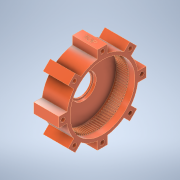
# Autodesk Inventor part: Gear_Box_Chasis_Lvl_1
Saved by Autodesk Inventor 2022 (Build 260153000, 153)
## iProperties
CustomPartVersion: 1
Created: 2022-04-22
Part Number: Gear_Box_Chasis_Lvl_1
Material: ABS Plastic
Document SubType Name: Modeling
Designer: Mlees
Categories: <?xml version="1.0" encoding="UTF-16"?> <MemberInstance><Categories><FamilyTemplate><FamilyTemplateParameter ValueType="xs:double" Id="1" ObjectReferenceKey="da_z" ObjectType="kUserParameterObject"/><FamilyTemplateParameter ValueType="xs:double" Id="2" ObjectReferenceKey="da_b" ObjectType="kUserParameterObject"/><FamilyTemplateParameter ValueType="xs:double" Id="3" ObjectReferenceKey="da_beta" ObjectType="kUserParameterObject"/><FamilyTemplateParameter ValueType="xs:double" Id="4" ObjectReferenceKey="da_da" ObjectType="kUserParameterObject"/><FamilyTemplateParameter ValueType="xs:double" Id="5" ObjectReferenceKey="da_aw" ObjectType="kUserParameterObject"/><FamilyTemplateParameter ValueType="xs:string" Id="6" ObjectReferenceKey="EAIAABAAAACIAQAAAAAAAIAAAAAAAAAA" ObjectType="83910656" SubObjectId="SurfaceGeometry"/></FamilyTemplate><ParamToTemplateMap><ParamToTemplate CategoryParameter="//CategoryParameter[@InternalName='046C89C9-8512-4d59-83FE-43B91F4F132A']" TemplateParameter="1"/><ParamToTemplate CategoryParameter="//CategoryParameter[@InternalName='2552DF32-E462-4b46-AEBF-C6C7768E72AC']" TemplateParameter="2"/><ParamToTemplate CategoryParameter="//CategoryParameter[@InternalName='C9EE641D-15FC-4fae-A226-E94C4372FDD7']" TemplateParameter="3"/><ParamToTemplate><ParamToTemplate CategoryParameter="//CategoryParameter[@InternalName='00B6519A-459B-49c7-AD84-2E56D39A5744']" ConstantValue="0.064200"/></ParamToTemplate><ParamToTemplate><ParamToTemplate CategoryParameter="//CategoryParameter[@InternalName='04B31F0E-C7A6-4894-AA32-9629BEFACF47']" ConstantValue="1.000000"/></ParamToTemplate><ParamToTemplate><ParamToTemplate CategoryParameter="//CategoryParameter[@InternalName='43CBEC2E-7847-49e7-A936-2F7889FCB2D9']" ConstantValue="0.250000"/></ParamToTemplate><ParamToTemplate><ParamToTemplate CategoryParameter="//CategoryParameter[@InternalName='B1EFC894-105D-4ebd-86BF-FA20ED196853']" ConstantValue="0.333500"/></ParamToTemplate><ParamToTemplate><ParamToTemplate CategoryParameter="//CategoryParameter[@InternalName='51175063-3D10-4879-93E8-6246FE8B403D']" ConstantValue="2060000000.000000"/></ParamToTemplate><ParamToTemplate><ParamToTemplate CategoryParameter="//CategoryParameter[@InternalName='A3A52E27-4454-46a9-B0BD-C932399B70AF']" ConstantValue="0.300000"/></ParamToTemplate><ParamToTemplate><ParamToTemplate CategoryParameter="//CategoryParameter[@InternalName='91B76062-C214-41d9-B1B9-14D2AB99603D']" ConstantValue="0.055000"/></ParamToTemplate><ParamToTemplate><ParamToTemplate CategoryParameter="//CategoryParameter[@InternalName='374E806E-8B8A-4dda-A9AA-1039D6500AD2']" ConstantValue="18.181818"/></ParamToTemplate><ParamToTemplate><ParamToTemplate CategoryParameter="//CategoryParameter[@InternalName='2D373A89-B862-43d6-8D0B-0CBF12AB9F6C']" ConstantValue="0.253073"/></ParamToTemplate><ParamToTemplate CategoryParameter="//CategoryParameter[@InternalName='37777632-D6A2-4fac-9D53-DB8ACD95C989']" TemplateParameter="4"/><ParamToTemplate CategoryParameter="//CategoryParameter[@InternalName='FD1017F1-B727-4f7e-9707-0F86F1FF9423']" TemplateParameter="5"/><ParamToTemplate><ParamToTemplate CategoryParameter="//CategoryParameter[@InternalName='9E1B4470-B2D3-4ff1-B813-535BB4CDF51A']" ConstantValue="3520000.000000"/></ParamToTemplate><ParamToTemplate><ParamToTemplate CategoryParameter="//CategoryParameter[@InternalName='F8452263-BFF6-458c-9FB1-07C4B99E95CD']" ConstantValue="11400000.000000"/></ParamToTemplate><ParamToTemplate><ParamToTemplate CategoryParameter="//CategoryParameter[@InternalName='3E3BB259-FD49-497f-8171-6EBC954A3479']" ConstantValue="2.000000"/></ParamToTemplate><ParamToTemplate CategoryParameter="//CategoryParameter[@InternalName='27C3BAF2-7550-4e4b-AE2C-0DB134B7D9B7']" TemplateParameter="6"/></ParamToTemplateMap><Category DisplayName="Gear" InternalName="DC85795E-93AB-48d5-8EEE-5A27447B64BD" Mnemonic="Gear"><CategoryParameter DisplayName="z" InternalName="046C89C9-8512-4d59-83FE-43B91F4F132A" Mnemonic="z"/><CategoryParameter DisplayName="b" InternalName="2552DF32-E462-4b46-AEBF-C6C7768E72AC" Mnemonic="b"/><CategoryParameter DisplayName="||b|" InternalName="C9EE641D-15FC-4fae-A226-E94C4372FDD7" Mnemonic="beta"/><CategoryParameter DisplayName="x" InternalName="00B6519A-459B-49c7-AD84-2E56D39A5744" Mnemonic="x"/><CategoryParameter DisplayName="a*" InternalName="04B31F0E-C7A6-4894-AA32-9629BEFACF47" Mnemonic="a"/><CategoryParameter DisplayName="c*" InternalName="43CBEC2E-7847-49e7-A936-2F7889FCB2D9" Mnemonic="c"/><CategoryParameter DisplayName="r|.f|*" InternalName="B1EFC894-105D-4ebd-86BF-FA20ED196853" Mnemonic="rf"/><CategoryParameter DisplayName="E" InternalName="51175063-3D10-4879-93E8-6246FE8B403D" Mnemonic="E"/><CategoryParameter DisplayName="||m|" InternalName="A3A52E27-4454-46a9-B0BD-C932399B70AF" Mnemonic="mi"/><Category DisplayName="SpurGear" InternalName="26C5A22E-A91E-4dfd-A3B3-23CCAFAE1764" Mnemonic="SpurGear"><CategoryParameter DisplayName="m" InternalName="91B76062-C214-41d9-B1B9-14D2AB99603D" Mnemonic="m"/><CategoryParameter DisplayName="P" InternalName="374E806E-8B8A-4dda-A9AA-1039D6500AD2" Mnemonic="PP"/><CategoryParameter DisplayName="||a|" InternalName="2D373A89-B862-43d6-8D0B-0CBF12AB9F6C" Mnemonic="alpha"/><CategoryParameter DisplayName="d|.a|" InternalName="37777632-D6A2-4fac-9D53-DB8ACD95C989" Mnemonic="da"/><CategoryParameter DisplayName="a|.w|" InternalName="FD1017F1-B727-4f7e-9707-0F86F1FF9423" Mnemonic="aw"/><CategoryParameter DisplayName="||s||.Flim|" InternalName="9E1B4470-B2D3-4ff1-B813-535BB4CDF51A" Mnemonic="sFlim"/><CategoryParameter DisplayName="||s||.Hlim|" InternalName="F8452263-BFF6-458c-9FB1-07C4B99E95CD" Mnemonic="sHlim"/><CategoryParameter DisplayName="type" InternalName="3E3BB259-FD49-497f-8171-6EBC954A3479" Mnemonic="type"/><Category DisplayName="InternalSpurGear" InternalName="7CF704F6-14A9-42f8-93CE-E71DF57C2B55" Mnemonic="InternalSpurGear"><CategoryParameter DisplayName="PitchDiameter" InternalName="27C3BAF2-7550-4e4b-AE2C-0DB134B7D9B7" Mnemonic="IDS_PITCHDIAM"/></Category></Category></Category></Categories></MemberInstance>
Density: 1.06 g/cm^3
Appearance: Smooth - Light Orange
Mass: 27.2175 g
Surface Area: 170.067 cm^2
Volume: 25.6769 cm^3
Author: Mlees
Autodesk Inventor part; units mm, degrees
ref_plane "YZ Plane" through (0, 0, 0) normal (1, 0, 0) x (0, 1, 0)
ref_plane "XZ Plane" through (0, 0, 0) normal (0, 1, 0) x (-1, 0, 0)
ref_plane "XY Plane" through (0, 0, 0) normal (0, 0, 1) x (1, 0, 0)
sketch "Sketch1" plane through (0, 0, 0) normal (0, 0, 1) x (1, 0, 0)
  circle A0 centre (0, 0) radius 28.6251
  dimension "d0" = 57.2502
  constraints: 1 centre point
  measures "d0" diameter of A0
extrude "Extrusion1" add sketch "Sketch1" along normal blind 8
ref_plane "Work Plane2" through (0, 0, 4) normal (0, 0, 1) x (1, 0, 0)
sketch "Sketch2" plane through (0, 0, 0) normal (0, 0, -1) x (-1, 0, 0)
  circle A0 centre (0, 0) radius 28.6251 projected
  circle A1 centre (0, 0) radius 25.3
  dimension "d3" = 50.6
  constraints: 1 centre point, 1 coincident
  measures "d3" diameter of A1
surface extrude "Pitch Diameter" sketch "Sketch2" against normal through all shown no curves A1
ref_plane "Work Plane8" through (0, 0, 0) normal (0.999417, 0.0341411, 0) x (0, 0, 1)
ref_plane "Work Plane9" through (0, 0, 0) normal (1, 0, 0) x (0, 1, 0)
spur gear teeth "Spur Gear" teeth 92 pitch diameter 50.6 tip diameter 49.6575 root diameter 52.0456 face width 8 start plane through (0, 0, 0) normal (0, 0, -1) x (-1, 0, 0)
sketch "Sketch3" plane through (0, 0, 8) normal (0, 0, 1) x (1, 0, 0)
  circle A0 centre (0, 0) radius 28.6251
  arc A1 (0.2222, -26.0219) -> (0.6358, -24.8206) centre (-6.3627, -23.0825) ccw projected
  circle A2 centre (0, 0) radius 26.0228
  constraints: 2 coincident, 1 centre point, 3 other
extrude "Extrusion2" add sketch "Sketch3" along normal blind 4
sketch "Sketch4" plane through (0, 0, 12) normal (0, 0, 1) x (1, 0, 0)
  circle A0 centre (0, 0) radius 8.5
  circle A1 centre (0, 0) radius 28.6251
  dimension "d55" = 17
  constraints: 2 centre point, 2 coincident
  measures "d55" diameter of A0
extrude "Extrusion3" add sketch "Sketch4" along normal blind 3
sketch "Sketch5" plane through (0, 0, 15) normal (0, 0, 1) x (1, 0, 0)
  circle A0 centre (0, 0) radius 8.5
  circle A1 centre (0, 0) radius 28.6251 projected
  circle A2 centre (0, 0) radius 28.6251
  line L0 (-4, 28.3442) -> (-4, 35)
  line L1 (4, 28.3442) -> (4, 35)
  line L2 (-4, 35) -> (4, 35)
  circle A3 centre (0, 31.6721) radius 1.7859
  line L3 (-27.5772, 21.9203) -> (-21.9203, 27.5772)
  circle A4 centre (-22.3956, 22.3956) radius 1.7859
  line L4 (-22.8708, 17.214) -> (-27.5772, 21.9203)
  line L5 (-17.214, 22.8708) -> (-21.9203, 27.5772)
  line L6 (-35, -4) -> (-35, 4)
  circle A5 centre (-31.6721, 0) radius 1.7859
  line L7 (-28.3442, -4) -> (-35, -4)
  line L8 (-28.3442, 4) -> (-35, 4)
  line L9 (-21.9203, -27.5772) -> (-27.5772, -21.9203)
  circle A6 centre (-22.3956, -22.3956) radius 1.7859
  line L10 (-17.214, -22.8708) -> (-21.9203, -27.5772)
  line L11 (-22.8708, -17.214) -> (-27.5772, -21.9203)
  line L12 (4, -35) -> (-4, -35)
  circle A7 centre (0, -31.6721) radius 1.7859
  line L13 (4, -28.3442) -> (4, -35)
  line L14 (-4, -28.3442) -> (-4, -35)
  line L15 (27.5772, -21.9203) -> (21.9203, -27.5772)
  circle A8 centre (22.3956, -22.3956) radius 1.7859
  line L16 (22.8708, -17.214) -> (27.5772, -21.9203)
  line L17 (17.214, -22.8708) -> (21.9203, -27.5772)
  line L18 (35, 4) -> (35, -4)
  circle A9 centre (31.6721, 0) radius 1.7859
  line L19 (28.3442, 4) -> (35, 4)
  line L20 (28.3442, -4) -> (35, -4)
  line L21 (21.9203, 27.5772) -> (27.5772, 21.9203)
  circle A10 centre (22.3956, 22.3956) radius 1.7859
  line L22 (17.214, 22.8708) -> (21.9203, 27.5772)
  line L23 (22.8708, 17.214) -> (27.5772, 21.9203)
  dimension "d63" = 3.5719
  dimension "d66" = 360
  constraints: 48 end point, 10 centre point, 2 coincident, 2 point on circle, 1 horizontal, 73 other
  measures "d63" diameter of A3
extrude "Extrusion4" add sketch "Sketch5" against normal up to surface (15 mm away) contours A1 L19 L18 L20 | A1 L22 L21 L23 | L16 L15 L17 A1 | A1 L0 L2 L1 | L13 L12 L14 A1 | A1 L4 L3 L5 | L10 L9 L11 A1 | A1 L7 L6 L8
sketch "Sketch6" plane through (0, 0, 0) normal (0, 0, -1) x (-1, 0, 0)
  circle A0 centre (0, 0) radius 26.0228
  arc A1 (-22.8708, 17.214) -> (-28.3442, 4) centre (0, 0) ccw projected
  arc A2 (-4, 28.3442) -> (-17.214, 22.8708) centre (0, 0) ccw projected
  line L0 (-4, 35) -> (4, 35) projected
  line L1 (-4, 28.3442) -> (-4, 35)
  line L2 (-4, 35) -> (4, 35)
  arc A3 (17.214, 22.8708) -> (4, 28.3442) centre (0, 0) ccw projected
  line L3 (4, 35) -> (4, 28.3442)
  circle A4 centre (0, 31.6721) radius 1.7859 projected
  circle A5 centre (0, 31.6721) radius 1.7859
  line L4 (-22.8708, 17.214) -> (-27.5772, 21.9203)
  line L5 (-27.5772, 21.9203) -> (-21.9203, 27.5772)
  line L6 (-21.9203, 27.5772) -> (-17.214, 22.8708)
  line L7 (-28.3442, -4) -> (-35, -4)
  line L8 (-35, -4) -> (-35, 4)
  line L9 (-35, 4) -> (-28.3442, 4)
  line L10 (-17.214, -22.8708) -> (-21.9203, -27.5772)
  line L11 (-21.9203, -27.5772) -> (-27.5772, -21.9203)
  line L12 (-27.5772, -21.9203) -> (-22.8708, -17.214)
  line L13 (4, -28.3442) -> (4, -35)
  line L14 (4, -35) -> (-4, -35)
  line L15 (-4, -35) -> (-4, -28.3442)
  line L16 (22.8708, -17.214) -> (27.5772, -21.9203)
  line L17 (27.5772, -21.9203) -> (21.9203, -27.5772)
  line L18 (21.9203, -27.5772) -> (17.214, -22.8708)
  line L19 (28.3442, 4) -> (35, 4)
  line L20 (35, 4) -> (35, -4)
  line L21 (35, -4) -> (28.3442, -4)
  line L22 (17.214, 22.8708) -> (21.9203, 27.5772)
  line L23 (21.9203, 27.5772) -> (27.5772, 21.9203)
  line L24 (27.5772, 21.9203) -> (22.8708, 17.214)
  arc A6 (17.214, 22.8708) -> (4, 28.3442) centre (0, 0) ccw
  arc A7 (28.3442, 4) -> (22.8708, 17.214) centre (0, 0) ccw
  arc A8 (22.8708, -17.214) -> (28.3442, -4) centre (0, 0) ccw
  arc A9 (4, -28.3442) -> (17.214, -22.8708) centre (0, 0) ccw
  arc A10 (-17.214, -22.8708) -> (-4, -28.3442) centre (0, 0) ccw
  arc A11 (-28.3442, -4) -> (-22.8708, -17.214) centre (0, 0) ccw
  arc A12 (-4, 28.3442) -> (-17.214, 22.8708) centre (0, 0) ccw
  arc A13 (-22.8708, 17.214) -> (-28.3442, 4) centre (0, 0) ccw
  circle A14 centre (-22.3956, 22.3956) radius 1.7859
  circle A15 centre (-31.6721, 0) radius 1.7859
  circle A16 centre (-22.3956, -22.3956) radius 1.7859
  circle A17 centre (0, -31.6721) radius 1.7859
  circle A18 centre (22.3956, -22.3956) radius 1.7859
  circle A19 centre (31.6721, 0) radius 1.7859
  circle A20 centre (22.3956, 22.3956) radius 1.7859
  point P0 (-17.214, 22.8708)
  point P1 (-28.3442, 4)
  dimension "d72" = 360
  dimension "d76" = 360
  constraints: 48 end point, 17 centre point, 17 point on circle, 3 coincident, 3 perpendicular, 74 other
extrude "Extrusion5" add sketch "Sketch6" along normal blind 5
sketch "Sketch7" plane through (0, 0, 12) normal (0, 0, -1) x (-1, 0, 0)
  arc A0 (-19.1693, 17.5989) -> (-18.5738, 16.4767) centre (-12.5267, 20.4051) ccw projected
  circle A1 centre (0, 0) radius 26.0228
  circle A2 centre (0, 0) radius 10
  dimension "d80" = 20
  constraints: 2 coincident, 1 centre point, 3 other
  measures "d80" diameter of A2
extrude "Extrusion6" add sketch "Sketch7" along normal blind 2
sketch "Sketch8" plane through (-4, 35, 15) normal (0, 1, 0) x (1, 0, 0)
  line L0 (5.763, 6.3839) -> (2.613, 6.3839)
  line L1 (2.613, 6.3839) -> (2.613, 5.2172)
  line L2 (2.613, 5.2172) -> (2.263, 5.2172)
  line L3 (2.263, 5.2172) -> (2.263, 7.9005)
  line L4 (2.263, 7.9005) -> (2.613, 7.9005)
  line L5 (2.613, 7.9005) -> (2.613, 6.7339)
  line L6 (2.613, 6.7339) -> (5.763, 6.7339)
  line L7 (5.763, 6.7339) -> (5.763, 6.3839)
  line L8 (5.7047, 6.4422) -> (2.5547, 6.4422)
  line L9 (2.5547, 6.4422) -> (2.5547, 5.2755)
  line L10 (2.5547, 5.2755) -> (2.3213, 5.2755)
  line L11 (2.3213, 5.2755) -> (2.3213, 7.8422)
  line L12 (2.3213, 7.8422) -> (2.5547, 7.8422)
  line L13 (2.5547, 7.8422) -> (2.5547, 6.6755)
  line L14 (2.5547, 6.6755) -> (5.7047, 6.6755)
  line L15 (5.7047, 6.6755) -> (5.7047, 6.4422)
  line L16 (5.6463, 6.5005) -> (2.4963, 6.5005)
  line L17 (2.4963, 6.5005) -> (2.4963, 5.3339)
  line L18 (2.4963, 5.3339) -> (2.3797, 5.3339)
  line L19 (2.3797, 5.3339) -> (2.3797, 7.7839)
  line L20 (2.3797, 7.7839) -> (2.4963, 7.7839)
  line L21 (2.4963, 7.7839) -> (2.4963, 6.6172)
  line L22 (2.4963, 6.6172) -> (5.6463, 6.6172)
  line L23 (5.6463, 6.6172) -> (5.6463, 6.5005)
  line L24 (5.588, 6.5589) -> (2.438, 6.5589)
  line L25 (2.438, 5.3922) -> (2.438, 7.7255)
  circle A0 centre (4.013, 9.8839) radius 1.75
  circle A1 centre (4.013, 9.8839) radius 1.6917
  circle A2 centre (4.013, 9.8839) radius 1.6333
  circle A3 centre (4.013, 9.8839) radius 1.575
  circle A4 centre (4.013, 9.8839) radius 1.5167
  circle A5 centre (4.013, 9.8839) radius 1.4583
  circle A6 centre (4.013, 9.8839) radius 1.4
  line L26 (5.763, 12.1005) -> (2.263, 12.1005)
  line L27 (2.263, 12.1005) -> (2.263, 13.7339)
  arc A7 (4.013, 13.7339) -> (2.263, 13.7339) centre (3.138, 13.7339) ccw
  line L28 (4.013, 13.7339) -> (4.013, 12.4505)
  line L29 (4.013, 12.4505) -> (5.763, 12.4505)
  line L30 (5.763, 12.4505) -> (5.763, 12.1005)
  line L31 (3.663, 12.4505) -> (2.613, 12.4505)
  line L32 (2.613, 12.4505) -> (2.613, 13.7339)
  arc A8 (3.663, 13.7339) -> (2.613, 13.7339) centre (3.138, 13.7339) ccw
  line L33 (3.663, 13.7339) -> (3.663, 12.4505)
  line L34 (3.7213, 12.3922) -> (2.5547, 12.3922)
  line L35 (2.5547, 12.3922) -> (2.5547, 13.7339)
  arc A9 (3.7213, 13.7339) -> (2.5547, 13.7339) centre (3.138, 13.7339) ccw
  line L36 (3.7213, 13.7339) -> (3.7213, 12.3922)
  line L37 (3.7797, 12.3339) -> (2.4963, 12.3339)
  line L38 (2.4963, 12.3339) -> (2.4963, 13.7339)
  arc A10 (3.7797, 13.7339) -> (2.4963, 13.7339) centre (3.138, 13.7339) ccw
  line L39 (3.7797, 13.7339) -> (3.7797, 12.3339)
  line L40 (5.7047, 12.1589) -> (2.3213, 12.1589)
  line L41 (2.3213, 12.1589) -> (2.3213, 13.7339)
  arc A11 (3.9547, 13.7339) -> (2.3213, 13.7339) centre (3.138, 13.7339) ccw
  line L42 (3.9547, 13.7339) -> (3.9547, 12.3922)
  line L43 (3.9547, 12.3922) -> (5.7047, 12.3922)
  line L44 (5.7047, 12.3922) -> (5.7047, 12.1589)
  line L45 (5.6463, 12.2172) -> (2.3797, 12.2172)
  line L46 (2.3797, 12.2172) -> (2.3797, 13.7339)
  arc A12 (3.8963, 13.7339) -> (2.3797, 13.7339) centre (3.138, 13.7339) ccw
  line L47 (3.8963, 13.7339) -> (3.8963, 12.3339)
  line L48 (3.8963, 12.3339) -> (5.6463, 12.3339)
  line L49 (5.6463, 12.3339) -> (5.6463, 12.2172)
  line L50 (5.588, 12.2755) -> (2.438, 12.2755)
  line L51 (2.438, 12.2755) -> (2.438, 13.7339)
  arc A13 (3.838, 13.7339) -> (2.438, 13.7339) centre (3.138, 13.7339) ccw
  line L52 (3.838, 13.7339) -> (3.838, 12.2755)
  point P0 (4, 15)
extrude "Extrusion7" cut sketch "Sketch8" against normal blind 1 contours L0 L1 L2 L3 L4 L5 L6 L7 | L8 L9 L10 L11 L12 L13 L14 L15 | L16 L17 L18 L19 L20 L21 L22 L23 | A0 | A1 | A2 | A3 | A4 | A5 | L26 L27 A7 L28 L29 L30 | L40 L41 A11 L42 L43 L44 | L45 L46 A12 L47 L48 L49
sketch "Sketch9" plane through (0, 0, 15) normal (0, 0, 1) x (1, 0, 0)
  circle A0 centre (0, 0) radius 21
  dimension "d85" = 42
  constraints: 1 centre point, 1 coincident
  measures "d85" diameter of A0
extrude "Extrusion8" cut sketch "Sketch9" against normal blind 2
equation "\"d0\" = 1.1 * da_df"
equation "\"d1\" = da_b"
equation "\"d3\" = da_d"
equation "\"d16\" = da_aw"
equation "\"d47\" = da_aw"
equation "\"d52\" = da_aw"
equation "\"da_df\" = 52.04562"
equation "\"da_b\" = 8"
equation "\"da_d\" = 50.6"
equation "\"da_aw\" = 16.271976"
body "Solid1"
body "Srf1"
